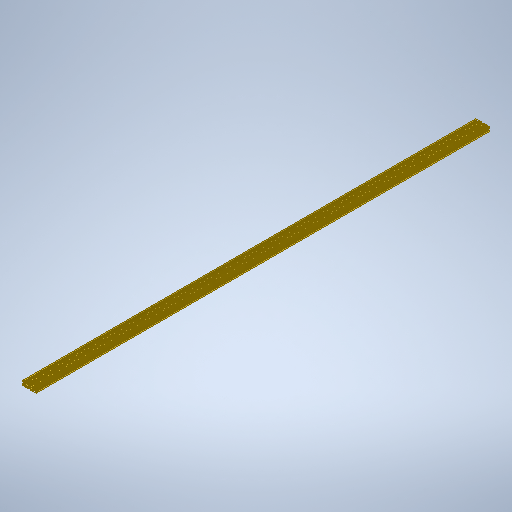
# Autodesk Inventor part: Perfil 20×40 6 rasgos_AST02004006
Saved by Autodesk Inventor 2025.2 (Build 292293000, 293)
## iProperties
Created: 2025-04-02
Part Number: Perfil 20×40 6 rasgos_AST02004006
Material: Ouro
Document SubType Name: Modeling
Designer: Gustavo Sousa
Density: 19.3 g/cm^3
Appearance: Metal quente 2400F
Author: Gustavo Sousa
Autodesk Inventor part; units mm, degrees
ref_plane "YZ Plane" through (0, 0, 0) normal (1, 0, 0) x (0, 1, 0)
ref_plane "XZ Plane" through (0, 0, 0) normal (0, 1, 0) x (-1, 0, 0)
ref_plane "XY Plane" through (0, 0, 0) normal (0, 0, 1) x (1, 0, 0)
sketch "Esboço2" plane through (0, 0, 0) normal (0, 0, 1) x (1, 0, 0)
  line L0 (-30, 10) -> (30, 10) construction
  line L1 (-30, 10) -> (-30, -10) construction
  line L2 (-3.1, 4) -> (3.1, 4) construction
  line L3 (-24, 3.1) -> (-24, -3.1) construction
  line L4 (-30, 10) -> (-10, 10) construction
  circle A0 centre (-20, 0) radius 2.5 construction
  line L5 (-20, 0) -> (-30, 10) construction
  line L6 (-30, 3.1) -> (-30, -3.1) construction
  line L7 (-30, 10) -> (-30, 3.1) construction
  line L8 (-30, 3.1) -> (-28, 3.1) construction
  line L9 (-28, 3.1) -> (-28, 7.1) construction
  line L10 (-28, 7.1) -> (-24, 3.1) construction
  line L11 (-24, 3.1) -> (-24, 0) construction
  line L12 (-23.1, 4) -> (-16.9, 4) construction
  line L13 (-23.1, 10) -> (-16.9, 10) construction
  line L14 (-23.1, 10) -> (-30, 10) construction
  line L15 (-23.1, 10) -> (-23.1, 8) construction
  line L16 (-27.1, 8) -> (-23.1, 8) construction
  line L17 (-27.1, 8) -> (-23.1, 4) construction
  line L18 (-16, 3.1) -> (-16, -3.1) construction
  line L19 (-16.9, 10) -> (-10, 10) construction
  line L20 (-16.9, 10) -> (-16.9, 8) construction
  line L21 (-16.9, 8) -> (-12.9, 8) construction
  line L22 (-20, 0) -> (-10, 10) construction
  line L23 (-16.9, 4) -> (-12.9, 8) construction
  line L24 (-16, 3.1) -> (-10.2313, 8.8687) construction
  line L25 (-10, 10) -> (-10, 9) construction
  arc A1 (-10, 9) -> (-10.2313, 8.8687) centre (-9.8777, 8.5152) ccw
  line L26 (-16, 3.1) -> (-16, 0) construction
  arc A2 (-25.8929, 8) -> (-26.2464, 7.1464) centre (-25.8929, 7.5) ccw
  arc A3 (-23.2464, 4.1464) -> (-22.8929, 4) centre (-22.8929, 4.5) ccw
  arc A4 (-17.1071, 4) -> (-16.7536, 4.1464) centre (-17.1071, 4.5) ccw
  arc A5 (-13.7536, 7.1464) -> (-14.1071, 8) centre (-14.1071, 7.5) ccw
  line L27 (-23.1, 10) -> (-23.6, 10) construction
  line L28 (-23.6, 10) -> (-23.6, 9.5)
  line L29 (-23.6, 9.5) -> (-23.1, 9.5)
  line L30 (-23.1, 9.5) -> (-23.1, 10) construction
  arc A6 (-29.5, 10) -> (-30, 9.5) centre (-29.5, 9.5) ccw
  line L31 (-30, 3.1) -> (-29.5, 3.1) construction
  line L32 (-29.5, 3.1) -> (-29.5, 3.6)
  line L33 (-29.5, 3.6) -> (-30, 3.6)
  line L34 (-30, 3.6) -> (-30, 3.1) construction
  line L35 (-30, 9.5) -> (-30, 3.6)
  line L36 (-29.5, 10) -> (-23.6, 10)
  line L37 (-23.1, 9.5) -> (-23.1, 8)
  line L38 (-23.1, 8) -> (-25.8929, 8)
  line L39 (-26.2464, 7.1464) -> (-23.2464, 4.1464)
  line L40 (-22.8929, 4) -> (-17.1071, 4)
  line L41 (-13.7536, 7.1464) -> (-16.7536, 4.1464)
  line L42 (-16.9, 8) -> (-14.1071, 8)
  line L43 (-16.9, 10) -> (-16.4, 10) construction
  line L44 (-16.4, 10) -> (-16.4, 9.5)
  line L45 (-16.4, 9.5) -> (-16.9, 9.5)
  line L46 (-16.9, 9.5) -> (-16.9, 10) construction
  line L47 (-16.9, 9.5) -> (-16.9, 8)
  line L48 (-16.4, 10) -> (-10, 10)
  arc A7 (-27.1464, 6.2464) -> (-28, 5.8929) centre (-27.5, 5.8929) ccw
  arc A8 (-24, 2.8929) -> (-24.1464, 3.2464) centre (-24.5, 2.8929) ccw
  line L49 (-29.5, 3.1) -> (-28, 3.1)
  line L50 (-28, 3.1) -> (-28, 5.8929)
  line L51 (-24.1464, 3.2464) -> (-27.1464, 6.2464)
  line L52 (-24, 2.8929) -> (-24, 0)
  arc A9 (-20, 2.5) -> (-22.5, 0) centre (-20, 0) ccw
  arc A10 (-17.5, 0) -> (-20, 2.5) centre (-20, 0) ccw
  line L53 (-17.5, 0) -> (-16, 0)
  line L54 (-24, 0) -> (-22.5, 0)
  arc A11 (-15.8536, 3.2464) -> (-16, 2.8929) centre (-15.5, 2.8929) ccw
  line L55 (-16, 2.8929) -> (-16, 0)
  line L56 (-15.8536, 3.2464) -> (-10.2313, 8.8687)
  line L57 (-10, 10) -> (10, 10) construction
  line L58 (-3.1, 10) -> (3.1, 10) construction
  circle A12 centre (0, 0) radius 2.5 construction
  line L59 (-10, 10) -> (-3.1, 10) construction
  line L60 (0, 0) -> (-10, 10) construction
  line L61 (-3.1, 10) -> (-3.1, 8) construction
  line L62 (-3.1, 8) -> (-7.1, 8) construction
  line L63 (-7.1, 8) -> (-3.1, 4) construction
  line L64 (-4, 3.1) -> (-4, -3.1) construction
  arc A13 (0, 2.5) -> (-2.5, 0) centre (0, 0) ccw
  line L65 (-9.7687, 8.8687) -> (-4, 3.1) construction
  arc A14 (-9.7687, 8.8687) -> (-10, 9) centre (-10.1223, 8.5152) ccw
  arc A15 (-4, 2.8929) -> (-4.1464, 3.2464) centre (-4.5, 2.8929) ccw
  line L66 (-9.7687, 8.8687) -> (-4.1464, 3.2464)
  line L67 (-4, 2.8929) -> (-4, 0)
  line L68 (-4, 0) -> (-2.5, 0)
  arc A16 (-5.8929, 8) -> (-6.2464, 7.1464) centre (-5.8929, 7.5) ccw
  arc A17 (-3.2464, 4.1464) -> (-2.8929, 4) centre (-2.8929, 4.5) ccw
  line L69 (-3.1, 10) -> (-3.6, 10) construction
  line L70 (-3.6, 10) -> (-3.6, 9.5)
  line L71 (-3.6, 9.5) -> (-3.1, 9.5)
  line L72 (-3.1, 9.5) -> (-3.1, 10) construction
  line L73 (-10, 10) -> (-3.6, 10)
  line L74 (-3.1, 9.5) -> (-3.1, 8)
  line L75 (-3.1, 8) -> (-5.8929, 8)
  line L76 (-6.2464, 7.1464) -> (-3.2464, 4.1464)
  line L77 (-2.8929, 4) -> (0, 4)
  line L78 (0, 4) -> (0, 2.5)
  point P0 (0, 10)
  point P1 (-30, 0)
  point P2 (-20, 10)
  point P3 (-30, 0)
  point P4 (-20, 4)
  point P5 (-20, 10)
  point P6 (-16.9, 9)
  point P7 (0, 10)
  point P8 (0, 10)
  dimension "d24" = 10
  dimension "d25" = 60
  dimension "d26" = 20
  dimension "d28" = 6.2
  dimension "d29" = 6
  dimension "d31" = 5
  dimension "d32" = 2
  dimension "d33" = 4
  dimension "d35" = 0.5
  dimension "d36" = 0.5
  dimension "d38" = 4
  dimension "d39" = 4
  constraints: 158 end point, 37 point on circle, 31 tangent, 24 equal length, 23 point on line, 18 centre point, 16 horizontal, 15 collinear, 14 parallel, 13 midpoint, 12 equal radius, 12 vertical, 9 horizontal alignment, 8 perpendicular, 7 vertical alignment, 6 coincident
  measures "d24" distance from line of point (0, 0) L0
  measures "d25" distance of L0.start L0.end
  measures "d26" distance of L0.start L1.end
  measures "d28" distance of L3.start L3.end
  measures "d29" distance between parallel lines of L1 L3
  measures "d31" diameter of A0
  measures "d32" distance between parallel lines of L1 L9
  measures "d33" distance from line of L5.start L18
  measures "d35" distance of L29.end L28.end
  measures "d36" radius of A6
  measures "d38" distance from line of point (0, 0) L2
  measures "d39" distance from line of point (0, 0) L64
extrude "Extrusão2" add sketch "Esboço2" along normal mid plane 2000
mirror "Espelhar5" about plane through (0, 0, 0) normal (0, 1, 0) of "Extrusão2"
mirror "Espelhar6" about plane through (0, 0, 0) normal (1, 0, 0) of "Extrusão2", "Espelhar5"
fillet "Arredondamento3" radius 1 2 edges at (-10, 9, 0) (10, 9, 0)
fillet "Arredondamento4" radius 1 2 edges at (-10, -9, 0) (10, -9, 0)
